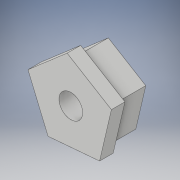
# Autodesk Inventor part: gearNotch
Saved by Autodesk Inventor 2019.1 (Build 231200000, 200)
## iProperties
Created: 2018-12-01
Part Number: gearNotch
Material: Generisch
Document SubType Name: Modeling
Designer: JochenAlt
Density: 1 g/cm^3
Appearance: Vorgabe
Author: JochenAlt
Autodesk Inventor part; units mm, degrees
ref_plane "YZ Plane" through (0, 0, 0) normal (1, 0, 0) x (0, 1, 0)
ref_plane "XZ Plane" through (0, 0, 0) normal (0, 1, 0) x (-1, 0, 0)
ref_plane "XY Plane" through (0, 0, 0) normal (0, 0, 1) x (1, 0, 0)
sketch "Skizze1" plane through (0, 0, 0) normal (0, 0, 1) x (1, 0, 0)
  circle A0 centre (0, 0) radius 4.2 construction
  line L0 (-0.3536, 4.1851) -> (3.871, 1.6296)
  line L1 (3.871, 1.6296) -> (2.746, -3.178)
  line L2 (2.746, -3.178) -> (-2.1739, -3.5937)
  line L3 (-2.1739, -3.5937) -> (-4.0895, 0.957)
  line L4 (-4.0895, 0.957) -> (-0.3536, 4.1851)
  circle A1 centre (0, 0) radius 5.5 construction
  line L5 (-0.4631, 5.4805) -> (5.0691, 2.134)
  line L6 (5.0691, 2.134) -> (3.596, -4.1616)
  line L7 (3.596, -4.1616) -> (-2.8467, -4.706)
  line L8 (-2.8467, -4.706) -> (-5.3553, 1.2532)
  line L9 (-5.3553, 1.2532) -> (-0.4631, 5.4805)
  circle A2 centre (0, 0) radius 1.75
  circle A3 centre (0, 0) radius 6.5 construction
  line L10 (-6.329, 1.481) -> (-0.5473, 6.4769)
  line L11 (-0.5473, 6.4769) -> (5.9908, 2.522)
  line L12 (5.9908, 2.522) -> (4.2498, -4.9183)
  line L13 (4.2498, -4.9183) -> (-3.3643, -5.5616)
  line L14 (-3.3643, -5.5616) -> (-6.329, 1.481)
  dimension "d6" = 8.4
  dimension "d7" = 11
  dimension "d9" = 13
  dimension "d8" = 3.5
  constraints: 30 end point, 7 coincident, 2 parallel, 1 centre point, 42 other
  measures "d8" diameter of A2
extrude "Extrusion1" add sketch "Skizze1" along normal blind 2.5 contours L5 L6 L7 L8 L9
extrude "Extrusion2" add sketch "Skizze1" along normal blind 1.5 from surface at 2.5 contours L0 L1 L2 L3 L4 | L5 L6 L7 L8 L9
extrude "Extrusion3" add sketch "Skizze1" along normal blind 2 from surface at 4 contours L0 L1 L2 L3 L4 | L5 L6 L7 L8 L9 | L10 L11 L12 L13 L14
